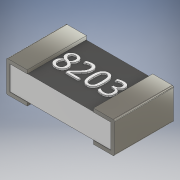
# Autodesk Inventor part: 21-1001
Saved by Autodesk Inventor 2018 (Build 220112000, 112)
## iProperties
Created: 2019-09-21
Part Number: 21-1001
Material: Copper
Document SubType Name: Modeling
Designer: Bradley
Density: 8.94 g/cm^3
Appearance: Smooth - White
Author: Bradley
Autodesk Inventor part; units mm, degrees
ref_plane "YZ Plane" through (0, 0, 0) normal (1, 0, 0) x (0, 1, 0)
ref_plane "XZ Plane" through (0, 0, 0) normal (0, 1, 0) x (-1, 0, 0)
ref_plane "XY Plane" through (0, 0, 0) normal (0, 0, 1) x (1, 0, 0)
sketch "Sketch1" plane through (0, 0, 0) normal (0, 1, 0) x (-1, 0, 0)
  line L0 (0.725, 0.175) -> (-0.725, 0.175)
  line L1 (-0.725, 0.175) -> (-0.725, -0.175)
  line L2 (-0.725, -0.175) -> (0.725, -0.175)
  line L3 (0.725, -0.175) -> (0.725, 0.175)
  line L4 (0.475, 0.175) -> (0.475, 0.225)
  line L5 (0.475, 0.225) -> (0.775, 0.225)
  line L6 (0.775, 0.225) -> (0.775, -0.225)
  line L7 (0.775, -0.225) -> (0.475, -0.225)
  line L8 (0.475, -0.225) -> (0.475, -0.175)
  line L9 (-0.475, 0.175) -> (-0.475, 0.225)
  line L10 (-0.475, 0.225) -> (-0.775, 0.225)
  line L11 (-0.775, 0.225) -> (-0.775, -0.225)
  line L12 (-0.775, -0.225) -> (-0.475, -0.225)
  line L13 (-0.475, -0.175) -> (-0.475, -0.225)
  line L14 (0.475, 0.175) -> (-0.475, 0.175)
  point P0 (0, 0)
  point P1 (0, 0.175)
  point P2 (0.725, 0)
  dimension "d0" = 1.55
  dimension "d1" = 0.05
  dimension "d2" = 0.05
  dimension "d3" = 0.45
  dimension "d4" = 0.3
  constraints: 30 end point, 12 point on line, 7 perpendicular, 3 collinear, 3 midpoint, 2 parallel, 1 horizontal, 1 horizontal alignment, 1 vertical, 1 vertical alignment
  measures "d0" distance between parallel lines of L11 L6
  measures "d1" distance of L7.end L8.end
  measures "d2" distance between parallel lines of L6 L3
  measures "d3" distance of L5.end L6.end
  measures "d4" distance of L6.end L7.end
extrude "Extrusion1" add sketch "Sketch1" along normal mid plane 0.85 contours L0 L4 L5 L6 L7 L8 L2 L3 | L0 L1 L2 L13 L12 L11 L10 L9
extrude "Extrusion2" add sketch "Sketch1" along normal mid plane 0.84 contours L3 L2 L1 L0
sketch "Sketch2" plane through (-0.475, -0.42, 0.175) normal (0, 0, 1) x (1, 0, 0)
  line L0 (0, 0) -> (0, 0.84) projected
  line L1 (0.95, 0) -> (0, 0) projected
  line L2 (0.95, 0) -> (0.95, 0.84) projected
  line L3 (0, 0.84) -> (0.95, 0.84) projected
  line L4 (0, 0.42) -> (0.95, 0.42) construction
  spline S0 degree 2 poles (0.1373, 0.2632) (0.115, 0.2632) (0.0782, 0.2766) (0.0654, 0.289) knots 0 0 0 1 2 2 2
  spline S1 degree 2 poles (0.0654, 0.289) (0.0527, 0.3011) (0.0396, 0.3342) (0.0396, 0.3529) knots 0 0 0 1 2 2 2
  spline S2 degree 2 poles (0.0396, 0.3529) (0.0396, 0.3772) (0.0656, 0.4181) (0.0904, 0.4302) knots 0 0 0 1 2 2 2
  line L5 (0.0904, 0.4302) -> (0.0904, 0.4314)
  spline S3 degree 2 poles (0.0904, 0.4314) (0.0683, 0.4443) (0.0469, 0.4749) (0.0469, 0.4978) knots 0 0 0 1 2 2 2
  spline S4 degree 2 poles (0.0469, 0.4978) (0.0469, 0.5316) (0.0979, 0.5768) (0.1373, 0.5768) knots 0 0 0 1 2 2 2
  spline S5 degree 2 poles (0.1373, 0.5768) (0.1782, 0.5768) (0.2275, 0.534) (0.2275, 0.5005) knots 0 0 0 1 2 2 2
  spline S6 degree 2 poles (0.2275, 0.5005) (0.2275, 0.4803) (0.2039, 0.4409) (0.1818, 0.4297) knots 0 0 0 1 2 2 2
  line L6 (0.1818, 0.4297) -> (0.1818, 0.4285)
  spline S7 degree 2 poles (0.1818, 0.4285) (0.2081, 0.4164) (0.235, 0.3813) (0.235, 0.3536) knots 0 0 0 1 2 2 2
  spline S8 degree 2 poles (0.235, 0.3536) (0.235, 0.3152) (0.1791, 0.2632) (0.1373, 0.2632) knots 0 0 0 1 2 2 2
  spline S9 degree 2 poles (0.1937, 0.3497) (0.1937, 0.3682) (0.1791, 0.3901) (0.1585, 0.4013) knots 0 0 0 1 2 2 2
  spline S10 degree 2 poles (0.1585, 0.4013) (0.1517, 0.4052) (0.1288, 0.4142) (0.1145, 0.42) knots 0 0 0 1 2 2 2
  spline S11 degree 2 poles (0.1145, 0.42) (0.0979, 0.4091) (0.0802, 0.3765) (0.0802, 0.3558) knots 0 0 0 1 2 2 2
  spline S12 degree 2 poles (0.0802, 0.3558) (0.0802, 0.3286) (0.113, 0.2931) (0.1378, 0.2931) knots 0 0 0 1 2 2 2
  spline S13 degree 2 poles (0.1378, 0.2931) (0.1631, 0.2931) (0.1937, 0.3235) (0.1937, 0.3497) knots 0 0 0 1 2 2 2
  spline S14 degree 2 poles (0.1881, 0.5) (0.1881, 0.5202) (0.1611, 0.5471) (0.1371, 0.5471) knots 0 0 0 1 2 2 2
  spline S15 degree 2 poles (0.1371, 0.5471) (0.1152, 0.5471) (0.0872, 0.5231) (0.0872, 0.5024) knots 0 0 0 1 2 2 2
  spline S16 degree 2 poles (0.0872, 0.5024) (0.0872, 0.4876) (0.1016, 0.4669) (0.1159, 0.4587) knots 0 0 0 1 2 2 2
  spline S17 degree 2 poles (0.1159, 0.4587) (0.122, 0.4553) (0.1478, 0.4433) (0.1582, 0.4399) knots 0 0 0 1 2 2 2
  spline S18 degree 2 poles (0.1582, 0.4399) (0.1757, 0.4533) (0.1881, 0.4818) (0.1881, 0.5) knots 0 0 0 1 2 2 2
  line L7 (0.4568, 0.27) -> (0.2718, 0.27)
  line L8 (0.2718, 0.27) -> (0.2718, 0.3125)
  spline S19 degree 2 poles (0.2718, 0.3125) (0.2917, 0.3313) (0.3272, 0.366) (0.3442, 0.3847) knots 0 0 0 1 2 2 2
  spline S20 degree 2 poles (0.3442, 0.3847) (0.3785, 0.4224) (0.4035, 0.4676) (0.4035, 0.4917) knots 0 0 0 1 2 2 2
  spline S21 degree 2 poles (0.4035, 0.4917) (0.4035, 0.5044) (0.3957, 0.5233) (0.3887, 0.5294) knots 0 0 0 1 2 2 2
  spline S22 degree 2 poles (0.3887, 0.5294) (0.3816, 0.5355) (0.3632, 0.5416) (0.352, 0.5416) knots 0 0 0 1 2 2 2
  spline S23 degree 2 poles (0.352, 0.5416) (0.3413, 0.5416) (0.3194, 0.5362) (0.3094, 0.5321) knots 0 0 0 1 2 2 2
  spline S24 degree 2 poles (0.3094, 0.5321) (0.3009, 0.5287) (0.2851, 0.5189) (0.2803, 0.5155) knots 0 0 0 1 2 2 2
  line L9 (0.2803, 0.5155) -> (0.2781, 0.5155)
  line L10 (0.2781, 0.5155) -> (0.2781, 0.5583)
  spline S25 degree 2 poles (0.2781, 0.5583) (0.2905, 0.5644) (0.335, 0.5763) (0.3549, 0.5763) knots 0 0 0 1 2 2 2
  spline S26 degree 2 poles (0.3549, 0.5763) (0.397, 0.5763) (0.4444, 0.5318) (0.4444, 0.4939) knots 0 0 0 1 2 2 2
  spline S27 degree 2 poles (0.4444, 0.4939) (0.4444, 0.4762) (0.4361, 0.4465) (0.4288, 0.4339) knots 0 0 0 1 2 2 2
  spline S28 degree 2 poles (0.4288, 0.4339) (0.4215, 0.4207) (0.4004, 0.395) (0.3887, 0.3826) knots 0 0 0 1 2 2 2
  spline S29 degree 2 poles (0.3887, 0.3826) (0.3697, 0.3619) (0.3233, 0.3176) (0.3094, 0.3048) knots 0 0 0 1 2 2 2
  line L11 (0.3094, 0.3048) -> (0.4568, 0.3048)
  line L12 (0.4568, 0.3048) -> (0.4568, 0.27)
  spline S30 degree 2 poles (0.6836, 0.42) (0.6836, 0.3393) (0.6367, 0.2637) (0.5878, 0.2637) knots 0 0 0 1 2 2 2
  spline S31 degree 2 poles (0.5878, 0.2637) (0.5382, 0.2637) (0.4918, 0.3407) (0.4918, 0.4198) knots 0 0 0 1 2 2 2
  spline S32 degree 2 poles (0.4918, 0.4198) (0.4918, 0.501) (0.5387, 0.5761) (0.5878, 0.5761) knots 0 0 0 1 2 2 2
  spline S33 degree 2 poles (0.5878, 0.5761) (0.6372, 0.5761) (0.6836, 0.4983) (0.6836, 0.42) knots 0 0 0 1 2 2 2
  spline S34 degree 2 poles (0.6321, 0.3286) (0.6379, 0.3434) (0.6427, 0.3891) (0.6427, 0.42) knots 0 0 0 1 2 2 2
  spline S35 degree 2 poles (0.6427, 0.42) (0.6427, 0.4509) (0.6379, 0.4963) (0.6318, 0.5117) knots 0 0 0 1 2 2 2
  spline S36 degree 2 poles (0.6318, 0.5117) (0.6257, 0.527) (0.6046, 0.5428) (0.5878, 0.5428) knots 0 0 0 1 2 2 2
  spline S37 degree 2 poles (0.5878, 0.5428) (0.571, 0.5428) (0.5494, 0.527) (0.5431, 0.5112) knots 0 0 0 1 2 2 2
  spline S38 degree 2 poles (0.5431, 0.5112) (0.537, 0.4959) (0.5326, 0.4492) (0.5326, 0.4198) knots 0 0 0 1 2 2 2
  spline S39 degree 2 poles (0.5326, 0.4198) (0.5326, 0.3882) (0.5365, 0.3459) (0.5428, 0.3293) knots 0 0 0 1 2 2 2
  spline S40 degree 2 poles (0.5428, 0.3293) (0.5487, 0.3138) (0.5703, 0.297) (0.5878, 0.297) knots 0 0 0 1 2 2 2
  spline S41 degree 2 poles (0.5878, 0.297) (0.6043, 0.297) (0.626, 0.3128) (0.6321, 0.3286) knots 0 0 0 1 2 2 2
  spline S42 degree 2 poles (0.803, 0.5416) (0.792, 0.5416) (0.7704, 0.5362) (0.7599, 0.5321) knots 0 0 0 1 2 2 2
  spline S43 degree 2 poles (0.7599, 0.5321) (0.7502, 0.5279) (0.7359, 0.5192) (0.7303, 0.5153) knots 0 0 0 1 2 2 2
  line L13 (0.7303, 0.5153) -> (0.7278, 0.5153)
  line L14 (0.7278, 0.5153) -> (0.7278, 0.5578)
  spline S44 degree 2 poles (0.7278, 0.5578) (0.741, 0.5649) (0.7859, 0.5763) (0.8061, 0.5763) knots 0 0 0 1 2 2 2
  spline S45 degree 2 poles (0.8061, 0.5763) (0.8265, 0.5763) (0.8569, 0.5681) (0.8693, 0.5593) knots 0 0 0 1 2 2 2
  spline S46 degree 2 poles (0.8693, 0.5593) (0.8825, 0.5498) (0.8961, 0.5224) (0.8961, 0.5039) knots 0 0 0 1 2 2 2
  spline S47 degree 2 poles (0.8961, 0.5039) (0.8961, 0.4791) (0.8635, 0.4416) (0.8406, 0.4368) knots 0 0 0 1 2 2 2
  line L15 (0.8406, 0.4368) -> (0.8406, 0.4339)
  spline S48 degree 2 poles (0.8406, 0.4339) (0.8501, 0.4319) (0.8718, 0.4232) (0.881, 0.4144) knots 0 0 0 1 2 2 2
  spline S49 degree 2 poles (0.881, 0.4144) (0.8902, 0.4059) (0.9019, 0.3787) (0.9019, 0.359) knots 0 0 0 1 2 2 2
  spline S50 degree 2 poles (0.9019, 0.359) (0.9019, 0.3388) (0.888, 0.3045) (0.8754, 0.2914) knots 0 0 0 1 2 2 2
  spline S51 degree 2 poles (0.8754, 0.2914) (0.8623, 0.2778) (0.8251, 0.2637) (0.8015, 0.2637) knots 0 0 0 1 2 2 2
  spline S52 degree 2 poles (0.8015, 0.2637) (0.7789, 0.2637) (0.7346, 0.2746) (0.7196, 0.2822) knots 0 0 0 1 2 2 2
  line L16 (0.7196, 0.2822) -> (0.7196, 0.3247)
  line L17 (0.7196, 0.3247) -> (0.7225, 0.3247)
  spline S53 degree 2 poles (0.7225, 0.3247) (0.7351, 0.3155) (0.7779, 0.2984) (0.7991, 0.2984) knots 0 0 0 1 2 2 2
  spline S54 degree 2 poles (0.7991, 0.2984) (0.8115, 0.2984) (0.8363, 0.3062) (0.8445, 0.3152) knots 0 0 0 1 2 2 2
  spline S55 degree 2 poles (0.8445, 0.3152) (0.8526, 0.3242) (0.8611, 0.3456) (0.8611, 0.3619) knots 0 0 0 1 2 2 2
  spline S56 degree 2 poles (0.8611, 0.3619) (0.8611, 0.3782) (0.8516, 0.3993) (0.8431, 0.4054) knots 0 0 0 1 2 2 2
  spline S57 degree 2 poles (0.8431, 0.4054) (0.8346, 0.4115) (0.8115, 0.4161) (0.7979, 0.4161) knots 0 0 0 1 2 2 2
  line L18 (0.7979, 0.4161) -> (0.7808, 0.4161)
  line L19 (0.7808, 0.4161) -> (0.7808, 0.4494)
  line L20 (0.7808, 0.4494) -> (0.7942, 0.4494)
  spline S58 degree 2 poles (0.7942, 0.4494) (0.8212, 0.4494) (0.8552, 0.4752) (0.8552, 0.4997) knots 0 0 0 1 2 2 2
  spline S59 degree 2 poles (0.8552, 0.4997) (0.8552, 0.5112) (0.8465, 0.5275) (0.8394, 0.5323) knots 0 0 0 1 2 2 2
  spline S60 degree 2 poles (0.8394, 0.5323) (0.8319, 0.5374) (0.8134, 0.5416) (0.803, 0.5416) knots 0 0 0 1 2 2 2
  point P0 (0.475, 0.42)
  constraints: 2 end point, 2 midpoint, 1 horizontal
extrude "Extrusion3" add sketch "Sketch2" along normal blind 0.02 contours S0 S1 S2 S3 S4 S5 S6 S7 S8 | L7 L8 S19 S20 S21 S22 S23 S24 L9 L10 S25 S26 S27 S28 S29 L11 L12 | S30 S31 S32 S33 | S42 S43 L13 L14 S44 S45 S46 S47 L15 S48 S49 S50 S51 S52 L16 L17 S53 S54 S55 S56 S57 L18 L19 L20 S58 S59 S60
fillet "Fillet1" radius 0.02 4 edges at (-0.775, 0, 0.225) (-0.775, 0, -0.225) (0.775, 0, 0.225) (0.775, 0, -0.225)
equation "\"d2\" = d1"
body "Solid1"
